Autodesk Fusion 360 part; units mm, degrees
(part 5 of 15)
  spline S28 degree 5 poles (37.7214, 5.5005) (37.7249, 5.5105) (37.7342, 5.5374) (37.7492, 5.5812) (37.7698, 5.6421) (37.7958, 5.72) (37.8238, 5.8051) (37.8515, 5.8904) (37.8788, 5.9759) (37.9057, 6.0616) (37.9322, 6.1474) (37.9584, 6.2335) (37.9843, 6.3197) (38.0098, 6.406) (38.035, 6.4926) (38.0599, 6.5793) (38.0844, 6.6662) (38.1085, 6.7532) (38.1324, 6.8404) (38.1559, 6.9278) (38.1791, 7.0153) (38.202, 7.103) (38.2246, 7.1908) (38.2469, 7.2788) (38.2688, 7.3669) (38.2905, 7.4552) (38.3118, 7.5436) (38.3328, 7.6322) (38.3536, 7.7209) (38.374, 7.8097) (38.3941, 7.8987) (38.414, 7.9878) (38.4335, 8.077) (38.4527, 8.1664) (38.4717, 8.2559) (38.4904, 8.3455) (38.5087, 8.4353) (38.5268, 8.5252) (38.5446, 8.6152) (38.5622, 8.7053) (38.5794, 8.7956) (38.5964, 8.886) (38.613, 8.9764) (38.6262, 9.0489) (38.6359, 9.1034) (38.6423, 9.1397) (38.6455, 9.1578) knots 0.405839 0.405839 0.405839 0.405839 0.405839 0.405839 0.414286 0.428571 0.442857 0.457143 0.471429 0.485714 0.5 0.514286 0.528571 0.542857 0.557143 0.571429 0.585714 0.6 0.614286 0.628571 0.642857 0.657143 0.671429 0.685714 0.7 0.714286 0.728571 0.742857 0.757143 0.771429 0.785714 0.8 0.814286 0.828571 0.842857 0.857143 0.871429 0.885714 0.9 0.914286 0.928571 0.942857 0.957143 0.971429 0.985714 1 1 1 1 1 1
  arc A29 (38.6455, 9.1578) -> (37.5327, 9.873) centre (-2.0032, -52.8695) ccw
  spline S29 degree 5 poles (37.5327, 9.873) (37.5175, 9.8625) (37.4872, 9.8416) (37.4417, 9.8101) (37.3812, 9.7681) (37.3058, 9.7153) (37.2307, 9.6624) (37.1557, 9.6092) (37.081, 9.5558) (37.0065, 9.5022) (36.9323, 9.4484) (36.8583, 9.3944) (36.7845, 9.3402) (36.711, 9.2858) (36.6377, 9.2311) (36.5646, 9.1763) (36.4918, 9.1212) (36.4192, 9.066) (36.3469, 9.0105) (36.2748, 8.9548) (36.203, 8.8989) (36.1314, 8.8427) (36.0601, 8.7864) (35.9891, 8.7298) (35.9183, 8.673) (35.8478, 8.616) (35.7776, 8.5587) (35.7076, 8.5013) (35.6379, 8.4436) (35.5685, 8.3856) (35.4994, 8.3275) (35.4305, 8.2691) (35.3619, 8.2105) (35.2937, 8.1516) (35.2257, 8.0925) (35.158, 8.0332) (35.0907, 7.9736) (35.0236, 7.9138) (34.9569, 7.8537) (34.8904, 7.7934) (34.8243, 7.7328) (34.7586, 7.672) (34.6985, 7.6159) (34.6517, 7.5719) (34.618, 7.54) (34.5974, 7.5204) (34.5898, 7.5131) knots -1 -1 -1 -1 -1 -1 -0.985714 -0.971429 -0.957143 -0.942857 -0.928571 -0.914286 -0.9 -0.885714 -0.871429 -0.857143 -0.842857 -0.828571 -0.814286 -0.8 -0.785714 -0.771429 -0.757143 -0.742857 -0.728571 -0.714286 -0.7 -0.685714 -0.671429 -0.657143 -0.642857 -0.628571 -0.614286 -0.6 -0.585714 -0.571429 -0.557143 -0.542857 -0.528571 -0.514286 -0.5 -0.485714 -0.471429 -0.457143 -0.442857 -0.428571 -0.414286 -0.405839 -0.405839 -0.405839 -0.405839 -0.405839 -0.405839
  arc A30 (34.5898, 7.5131) -> (33.4562, 8.1857) centre (-2.0032, -52.8695) ccw
  spline S30 degree 5 poles (33.4562, 8.1857) (33.4589, 8.1959) (33.4662, 8.2234) (33.4781, 8.2682) (33.4943, 8.3304) (33.5147, 8.41) (33.5366, 8.4969) (33.5581, 8.5839) (33.5792, 8.6711) (33.5999, 8.7585) (33.6203, 8.846) (33.6403, 8.9337) (33.6599, 9.0215) (33.6792, 9.1095) (33.6982, 9.1976) (33.7168, 9.2859) (33.735, 9.3743) (33.7529, 9.4629) (33.7705, 9.5515) (33.7877, 9.6404) (33.8046, 9.7293) (33.8212, 9.8184) (33.8375, 9.9076) (33.8534, 9.997) (33.869, 10.0864) (33.8843, 10.176) (33.8993, 10.2657) (33.9139, 10.3556) (33.9283, 10.4455) (33.9423, 10.5356) (33.956, 10.6257) (33.9695, 10.716) (33.9826, 10.8065) (33.9954, 10.897) (34.0079, 10.9876) (34.0202, 11.0783) (34.0321, 11.1692) (34.0437, 11.2601) (34.0551, 11.3512) (34.0661, 11.4423) (34.0769, 11.5336) (34.0873, 11.6249) (34.0975, 11.7164) (34.1054, 11.7896) (34.1113, 11.8446) (34.1151, 11.8813) (34.117, 11.8996) knots 0.405839 0.405839 0.405839 0.405839 0.405839 0.405839 0.414286 0.428571 0.442857 0.457143 0.471429 0.485714 0.5 0.514286 0.528571 0.542857 0.557143 0.571429 0.585714 0.6 0.614286 0.628571 0.642857 0.657143 0.671429 0.685714 0.7 0.714286 0.728571 0.742857 0.757143 0.771429 0.785714 0.8 0.814286 0.828571 0.842857 0.857143 0.871429 0.885714 0.9 0.914286 0.928571 0.942857 0.957143 0.971429 0.985714 1 1 1 1 1 1
  arc A31 (34.117, 11.8996) -> (32.956, 12.5336) centre (-2.0032, -52.8695) ccw
  spline S31 degree 5 poles (32.956, 12.5336) (32.9416, 12.5221) (32.9128, 12.499) (32.8697, 12.4644) (32.8124, 12.4182) (32.7409, 12.3601) (32.6697, 12.3019) (32.5988, 12.2436) (32.5281, 12.185) (32.4576, 12.1262) (32.3874, 12.0672) (32.3174, 12.0081) (32.2477, 11.9488) (32.1782, 11.8892) (32.109, 11.8295) (32.04, 11.7696) (31.9713, 11.7095) (31.9029, 11.6492) (31.8347, 11.5887) (31.7668, 11.528) (31.6992, 11.4671) (31.6318, 11.406) (31.5647, 11.3447) (31.4979, 11.2832) (31.4313, 11.2215) (31.365, 11.1596) (31.2991, 11.0975) (31.2334, 11.0352) (31.168, 10.9726) (31.1029, 10.9099) (31.0381, 10.847) (30.9736, 10.7838) (30.9093, 10.7204) (30.8455, 10.6569) (30.7819, 10.5931) (30.7186, 10.5291) (30.6557, 10.4648) (30.593, 10.4004) (30.5308, 10.3357) (30.4688, 10.2708) (30.4072, 10.2057) (30.3459, 10.1403) (30.29, 10.0801) (30.2465, 10.0328) (30.2152, 9.9986) (30.196, 9.9776) (30.1889, 9.9698) knots -1 -1 -1 -1 -1 -1 -0.985714 -0.971429 -0.957143 -0.942857 -0.928571 -0.914286 -0.9 -0.885714 -0.871429 -0.857143 -0.842857 -0.828571 -0.814286 -0.8 -0.785714 -0.771429 -0.757143 -0.742857 -0.728571 -0.714286 -0.7 -0.685714 -0.671429 -0.657143 -0.642857 -0.628571 -0.614286 -0.6 -0.585714 -0.571429 -0.557143 -0.542857 -0.528571 -0.514286 -0.5 -0.485714 -0.471429 -0.457143 -0.442857 -0.428571 -0.414286 -0.405839 -0.405839 -0.405839 -0.405839 -0.405839 -0.405839
  arc A32 (30.1889, 9.9698) -> (29.0102, 10.5598) centre (-2.0032, -52.8695) ccw
  spline S32 degree 5 poles (29.0102, 10.5598) (29.0122, 10.5702) (29.0175, 10.5981) (29.0261, 10.6436) (29.0379, 10.7068) (29.0526, 10.7877) (29.0682, 10.8759) (29.0834, 10.9643) (29.0982, 11.0528) (29.1127, 11.1414) (29.1268, 11.2301) (29.1405, 11.319) (29.1538, 11.408) (29.1668, 11.4972) (29.1794, 11.5864) (29.1916, 11.6758) (29.2035, 11.7653) (29.2151, 11.8549) (29.2263, 11.9446) (29.2371, 12.0344) (29.2477, 12.1243) (29.2578, 12.2144) (29.2677, 12.3045) (29.2772, 12.3948) (29.2864, 12.4851) (29.2952, 12.5756) (29.3038, 12.6661) (29.312, 12.7568) (29.3199, 12.8475) (29.3275, 12.9383) (29.3347, 13.0293) (29.3417, 13.1203) (29.3483, 13.2114) (29.3546, 13.3026) (29.3607, 13.3939) (29.3664, 13.4853) (29.3718, 13.5767) (29.3769, 13.6683) (29.3817, 13.7599) (29.3862, 13.8516) (29.3905, 13.9434) (29.3944, 14.0353) (29.398, 14.1272) (29.4007, 14.2009) (29.4026, 14.2561) (29.4038, 14.293) (29.4044, 14.3114) knots 0.405839 0.405839 0.405839 0.405839 0.405839 0.405839 0.414286 0.428571 0.442857 0.457143 0.471429 0.485714 0.5 0.514286 0.528571 0.542857 0.557143 0.571429 0.585714 0.6 0.614286 0.628571 0.642857 0.657143 0.671429 0.685714 0.7 0.714286 0.728571 0.742857 0.757143 0.771429 0.785714 0.8 0.814286 0.828571 0.842857 0.857143 0.871429 0.885714 0.9 0.914286 0.928571 0.942857 0.957143 0.971429 0.985714 1 1 1 1 1 1
  arc A33 (29.4044, 14.3114) -> (28.2011, 14.8609) centre (-2.0032, -52.8695) ccw
  spline S33 degree 5 poles (28.2011, 14.8609) (28.1876, 14.8484) (28.1605, 14.8234) (28.12, 14.7858) (28.0661, 14.7355) (27.999, 14.6726) (27.9321, 14.6094) (27.8655, 14.5461) (27.7992, 14.4827) (27.7331, 14.419) (27.6672, 14.3552) (27.6017, 14.2912) (27.5363, 14.227) (27.4713, 14.1627) (27.4065, 14.0982) (27.342, 14.0335) (27.2778, 13.9687) (27.2138, 13.9036) (27.1501, 13.8384) (27.0867, 13.773) (27.0236, 13.7075) (26.9607, 13.6417) (26.8982, 13.5758) (26.8359, 13.5097) (26.7739, 13.4434) (26.7122, 13.3769) (26.6509, 13.3102) (26.5898, 13.2434) (26.529, 13.1764) (26.4685, 13.1092) (26.4084, 13.0418) (26.3486, 12.9742) (26.289, 12.9064) (26.2298, 12.8384) (26.171, 12.7702) (26.1124, 12.7019) (26.0542, 12.6333) (25.9964, 12.5646) (25.9389, 12.4956) (25.8817, 12.4264) (25.8249, 12.3571) (25.7684, 12.2875) (25.7169, 12.2234) (25.6769, 12.1732) (25.6481, 12.1369) (25.6305, 12.1145) (25.624, 12.1062) knots -1 -1 -1 -1 -1 -1 -0.985714 -0.971429 -0.957143 -0.942857 -0.928571 -0.914286 -0.9 -0.885714 -0.871429 -0.857143 -0.842857 -0.828571 -0.814286 -0.8 -0.785714 -0.771429 -0.757143 -0.742857 -0.728571 -0.714286 -0.7 -0.685714 -0.671429 -0.657143 -0.642857 -0.628571 -0.614286 -0.6 -0.585714 -0.571429 -0.557143 -0.542857 -0.528571 -0.514286 -0.5 -0.485714 -0.471429 -0.457143 -0.442857 -0.428571 -0.414286 -0.405839 -0.405839 -0.405839 -0.405839 -0.405839 -0.405839
  arc A34 (25.624, 12.1062) -> (24.4062, 12.6106) centre (-2.0032, -52.8695) ccw
  spline S34 degree 5 poles (24.4062, 12.6106) (24.4074, 12.6211) (24.4108, 12.6494) (24.4161, 12.6954) (24.4233, 12.7593) (24.4322, 12.841) (24.4415, 12.9301) (24.4504, 13.0193) (24.4588, 13.1086) (24.4669, 13.1981) (24.4746, 13.2876) (24.482, 13.3772) (24.4889, 13.467) (24.4955, 13.5568) (24.5017, 13.6467) (24.5075, 13.7367) (24.513, 13.8268) (24.5182, 13.917) (24.5229, 14.0073) (24.5273, 14.0977) (24.5314, 14.1881) (24.5352, 14.2787) (24.5385, 14.3693) (24.5416, 14.46) (24.5443, 14.5508) (24.5467, 14.6416) (24.5488, 14.7326) (24.5505, 14.8236) (24.5519, 14.9146) (24.553, 15.0058) (24.5537, 15.097) (24.5542, 15.1883) (24.5543, 15.2796) (24.5541, 15.3711) (24.5536, 15.4625) (24.5528, 15.5541) (24.5516, 15.6457) (24.5502, 15.7374) (24.5485, 15.8291) (24.5464, 15.9209) (24.5441, 16.0128) (24.5415, 16.1047) (24.5385, 16.1967) (24.536, 16.2703) (24.5339, 16.3256) (24.5324, 16.3624) (24.5317, 16.3808) knots 0.405839 0.405839 0.405839 0.405839 0.405839 0.405839 0.414286 0.428571 0.442857 0.457143 0.471429 0.485714 0.5 0.514286 0.528571 0.542857 0.557143 0.571429 0.585714 0.6 0.614286 0.628571 0.642857 0.657143 0.671429 0.685714 0.7 0.714286 0.728571 0.742857 0.757143 0.771429 0.785714 0.8 0.814286 0.828571 0.842857 0.857143 0.871429 0.885714 0.9 0.914286 0.928571 0.942857 0.957143 0.971429 0.985714 1 1 1 1 1 1
  arc A35 (24.5317, 16.3808) -> (23.2923, 16.8431) centre (-2.0032, -52.8695) ccw
  spline S35 degree 5 poles (23.2923, 16.8431) (23.2797, 16.8296) (23.2545, 16.8027) (23.2168, 16.7623) (23.1666, 16.7084) (23.1041, 16.6408) (23.042, 16.5731) (22.98, 16.5052) (22.9184, 16.4371) (22.857, 16.3689) (22.7959, 16.3006) (22.735, 16.2321) (22.6745, 16.1634) (22.6142, 16.0946) (22.5542, 16.0256) (22.4944, 15.9565) (22.435, 15.8872) (22.3758, 15.8178) (22.3169, 15.7482) (22.2584, 15.6785) (22.2001, 15.6086) (22.1421, 15.5385) (22.0844, 15.4683) (22.027, 15.3979) (21.9699, 15.3274) (21.9131, 15.2566) (21.8566, 15.1858) (21.8005, 15.1148) (21.7447, 15.0436) (21.6891, 14.9722) (21.634, 14.9007) (21.5791, 14.829) (21.5246, 14.7571) (21.4704, 14.6851) (21.4165, 14.6129) (21.363, 14.5405) (21.3098, 14.468) (21.257, 14.3953) (21.2046, 14.3224) (21.1525, 14.2494) (21.1008, 14.1761) (21.0494, 14.1027) (21.0026, 14.0351) (20.9663, 13.9821) (20.9402, 13.9439) (20.9242, 13.9203) (20.9183, 13.9116) knots -1 -1 -1 -1 -1 -1 -0.985714 -0.971429 -0.957143 -0.942857 -0.928571 -0.914286 -0.9 -0.885714 -0.871429 -0.857143 -0.842857 -0.828571 -0.814286 -0.8 -0.785714 -0.771429 -0.757143 -0.742857 -0.728571 -0.714286 -0.7 -0.685714 -0.671429 -0.657143 -0.642857 -0.628571 -0.614286 -0.6 -0.585714 -0.571429 -0.557143 -0.542857 -0.528571 -0.514286 -0.5 -0.485714 -0.471429 -0.457143 -0.442857 -0.428571 -0.414286 -0.405839 -0.405839 -0.405839 -0.405839 -0.405839 -0.405839
  arc A36 (20.9183, 13.9116) -> (19.6676, 14.3278) centre (-2.0032, -52.8695) ccw
  spline S36 degree 5 poles (19.6676, 14.3278) (19.6681, 14.3384) (19.6694, 14.3668) (19.6715, 14.4131) (19.6741, 14.4773) (19.6771, 14.5594) (19.68, 14.649) (19.6825, 14.7386) (19.6846, 14.8283) (19.6863, 14.9181) (19.6876, 15.0079) (19.6885, 15.0979) (19.689, 15.1879) (19.6892, 15.2779) (19.689, 15.3681) (19.6884, 15.4583) (19.6874, 15.5486) (19.6861, 15.6389) (19.6844, 15.7293) (19.6824, 15.8197) (19.68, 15.9102) (19.6772, 16.0008) (19.6742, 16.0914) (19.6707, 16.1821) (19.667, 16.2729) (19.6629, 16.3637) (19.6584, 16.4545) (19.6537, 16.5454) (19.6486, 16.6363) (19.6431, 16.7273) (19.6374, 16.8184) (19.6313, 16.9095) (19.6249, 17.0006) (19.6182, 17.0918) (19.6112, 17.183) (19.6038, 17.2742) (19.5962, 17.3655) (19.5882, 17.4569) (19.5799, 17.5483) (19.5713, 17.6397) (19.5625, 17.7312) (19.5533, 17.8226) (19.5438, 17.9142) (19.536, 17.9874) (19.53, 18.0424) (19.5259, 18.079) (19.5238, 18.0974) knots 0.405839 0.405839 0.405839 0.405839 0.405839 0.405839 0.414286 0.428571 0.442857 0.457143 0.471429 0.485714 0.5 0.514286 0.528571 0.542857 0.557143 0.571429 0.585714 0.6 0.614286 0.628571 0.642857 0.657143 0.671429 0.685714 0.7 0.714286 0.728571 0.742857 0.757143 0.771429 0.785714 0.8 0.814286 0.828571 0.842857 0.857143 0.871429 0.885714 0.9 0.914286 0.928571 0.942857 0.957143 0.971429 0.985714 1 1 1 1 1 1
  arc A37 (19.5238, 18.0974) -> (18.2546, 18.47) centre (-2.0032, -52.8695) ccw
  spline S37 degree 5 poles (18.2546, 18.47) (18.243, 18.4557) (18.2198, 18.4271) (18.185, 18.3841) (18.1388, 18.3267) (18.0814, 18.2548) (18.0242, 18.1828) (17.9672, 18.1107) (17.9106, 18.0384) (17.8542, 17.966) (17.7982, 17.8935) (17.7424, 17.8208) (17.6868, 17.748) (17.6316, 17.6751) (17.5767, 17.602) (17.522, 17.5288) (17.4677, 17.4555) (17.4136, 17.382) (17.3598, 17.3084) (17.3064, 17.2346) (17.2532, 17.1607) (17.2004, 17.0867) (17.1478, 17.0126) (17.0956, 16.9383) (17.0437, 16.8638) (16.9921, 16.7892) (16.9409, 16.7145) (16.8899, 16.6397) (16.8393, 16.5647) (16.789, 16.4895) (16.7391, 16.4143) (16.6895, 16.3388) (16.6402, 16.2633) (16.5913, 16.1876) (16.5427, 16.1117) (16.4945, 16.0357) (16.4466, 15.9596) (16.3991, 15.8833) (16.352, 15.8068) (16.3053, 15.7303) (16.2589, 15.6535) (16.213, 15.5766) (16.1711, 15.5059) (16.1386, 15.4504) (16.1153, 15.4104) (16.101, 15.3858) (16.0958, 15.3766) knots -1 -1 -1 -1 -1 -1 -0.985714 -0.971429 -0.957143 -0.942857 -0.928571 -0.914286 -0.9 -0.885714 -0.871429 -0.857143 -0.842857 -0.828571 -0.814286 -0.8 -0.785714 -0.771429 -0.757143 -0.742857 -0.728571 -0.714286 -0.7 -0.685714 -0.671429 -0.657143 -0.642857 -0.628571 -0.614286 -0.6 -0.585714 -0.571429 -0.557143 -0.542857 -0.528571 -0.514286 -0.5 -0.485714 -0.471429 -0.457143 -0.442857 -0.428571 -0.414286 -0.405839 -0.405839 -0.405839 -0.405839 -0.405839 -0.405839
  arc A38 (16.0958, 15.3766) -> (14.8186, 15.7026) centre (-2.0032, -52.8695) ccw
  spline S38 degree 5 poles (14.8186, 15.7026) (14.8183, 15.7132) (14.8176, 15.7416) (14.8163, 15.7879) (14.8144, 15.8522) (14.8116, 15.9343) (14.8081, 16.0238) (14.8041, 16.1134) (14.7998, 16.203) (14.7951, 16.2927) (14.79, 16.3824) (14.7845, 16.4722) (14.7786, 16.562) (14.7723, 16.6518) (14.7657, 16.7417) (14.7586, 16.8317) (14.7513, 16.9216) (14.7435, 17.0116) (14.7354, 17.1017) (14.7269, 17.1918) (14.718, 17.2819) (14.7089, 17.372) (14.6993, 17.4622) (14.6894, 17.5524) (14.6792, 17.6426) (14.6686, 17.7329) (14.6577, 17.8232) (14.6465, 17.9135) (14.6349, 18.0039) (14.623, 18.0942) (14.6108, 18.1846) (14.5982, 18.2751) (14.5853, 18.3655) (14.5721, 18.456) (14.5586, 18.5465) (14.5448, 18.637) (14.5306, 18.7275) (14.5162, 18.818) (14.5014, 18.9086) (14.4863, 18.9992) (14.4709, 19.0897) (14.4552, 19.1804) (14.4392, 19.271) (14.4262, 19.3435) (14.4163, 19.3979) (14.4096, 19.4341) (14.4063, 19.4523) knots 0.405839 0.405839 0.405839 0.405839 0.405839 0.405839 0.414286 0.428571 0.442857 0.457143 0.471429 0.485714 0.5 0.514286 0.528571 0.542857 0.557143 0.571429 0.585714 0.6 0.614286 0.628571 0.642857 0.657143 0.671429 0.685714 0.7 0.714286 0.728571 0.742857 0.757143 0.771429 0.785714 0.8 0.814286 0.828571 0.842857 0.857143 0.871429 0.885714 0.9 0.914286 0.928571 0.942857 0.957143 0.971429 0.985714 1 1 1 1 1 1
  arc A39 (14.4063, 19.4523) -> (13.1137, 19.7334) centre (-2.0032, -52.8695) ccw
  spline S39 degree 5 poles (13.1137, 19.7334) (13.1031, 19.7183) (13.082, 19.6881) (13.0504, 19.6428) (13.0084, 19.5822) (12.9562, 19.5064) (12.9043, 19.4305) (12.8527, 19.3545) (12.8014, 19.2784) (12.7503, 19.2022) (12.6995, 19.1258) (12.6491, 19.0493) (12.5989, 18.9728) (12.549, 18.8961) (12.4994, 18.8193) (12.4501, 18.7423) (12.4011, 18.6653) (12.3524, 18.5882) (12.3041, 18.5109) (12.256, 18.4335) (12.2083, 18.356) (12.1608, 18.2784) (12.1137, 18.2007) (12.0669, 18.1229) (12.0205, 18.0449) (11.9743, 17.9669) (11.9285, 17.8887) (11.883, 17.8104) (11.8379, 17.732) (11.7931, 17.6534) (11.7487, 17.5748) (11.7046, 17.496) (11.6608, 17.4171) (11.6174, 17.3381) (11.5744, 17.259) (11.5317, 17.1798) (11.4894, 17.1004) (11.4475, 17.0209) (11.406, 16.9413) (11.3648, 16.8616) (11.324, 16.7817) (11.2837, 16.7018) (11.2469, 16.6282) (11.2185, 16.5706) (11.1981, 16.529) (11.1856, 16.5034) (11.181, 16.4939) knots -1 -1 -1 -1 -1 -1 -0.985714 -0.971429 -0.957143 -0.942857 -0.928571 -0.914286 -0.9 -0.885714 -0.871429 -0.857143 -0.842857 -0.828571 -0.814286 -0.8 -0.785714 -0.771429 -0.757143 -0.742857 -0.728571 -0.714286 -0.7 -0.685714 -0.671429 -0.657143 -0.642857 -0.628571 -0.614286 -0.6 -0.585714 -0.571429 -0.557143 -0.542857 -0.528571 -0.514286 -0.5 -0.485714 -0.471429 -0.457143 -0.442857 -0.428571 -0.414286 -0.405839 -0.405839 -0.405839 -0.405839 -0.405839 -0.405839
  arc A40 (11.181, 16.4939) -> (9.8838, 16.7279) centre (-2.0032, -52.8695) ccw
  spline S40 degree 5 poles (9.8838, 16.7279) (9.8828, 16.7385) (9.8801, 16.7668) (9.8755, 16.8129) (9.869, 16.8768) (9.8603, 16.9586) (9.8504, 17.0476) (9.8401, 17.1367) (9.8294, 17.2257) (9.8183, 17.3149) (9.8068, 17.404) (9.7949, 17.4931) (9.7827, 17.5823) (9.77, 17.6714) (9.7569, 17.7606) (9.7435, 17.8498) (9.7297, 17.9391) (9.7156, 18.0283) (9.701, 18.1175) (9.6861, 18.2068) (9.6709, 18.296) (9.6553, 18.3853) (9.6394, 18.4745) (9.6231, 18.5638) (9.6064, 18.6531) (9.5894, 18.7424) (9.5721, 18.8317) (9.5545, 18.921) (9.5365, 19.0102) (9.5181, 19.0995) (9.4995, 19.1888) (9.4805, 19.2781) (9.4612, 19.3674) (9.4416, 19.4567) (9.4217, 19.546) (9.4014, 19.6353) (9.3808, 19.7246) (9.3599, 19.8138) (9.3387, 19.9031) (9.3172, 19.9924) (9.2954, 20.0817) (9.2733, 20.1709) (9.2509, 20.2602) (9.2327, 20.3316) (9.219, 20.3851) (9.2097, 20.4208) (9.2051, 20.4386) knots 0.405839 0.405839 0.405839 0.405839 0.405839 0.405839 0.414286 0.428571 0.442857 0.457143 0.471429 0.485714 0.5 0.514286 0.528571 0.542857 0.557143 0.571429 0.585714 0.6 0.614286 0.628571 0.642857 0.657143 0.671429 0.685714 0.7 0.714286 0.728571 0.742857 0.757143 0.771429 0.785714 0.8 0.814286 0.828571 0.842857 0.857143 0.871429 0.885714 0.9 0.914286 0.928571 0.942857 0.957143 0.971429 0.985714 1 1 1 1 1 1
  arc A41 (9.2051, 20.4386) -> (7.8958, 20.6269) centre (-2.0032, -52.8695) ccw
  spline S41 degree 5 poles (7.8958, 20.6269) (7.8863, 20.6111) (7.8674, 20.5794) (7.8391, 20.5319) (7.8015, 20.4685) (7.7549, 20.3892) (7.7085, 20.3098) (7.6624, 20.2303) (7.6167, 20.1507) (7.5712, 20.071) (7.526, 19.9913) (7.4811, 19.9114) (7.4365, 19.8314) (7.3922, 19.7514) (7.3482, 19.6712) (7.3046, 19.591) (7.2612, 19.5106) (7.2181, 19.4302) (7.1754, 19.3497) (7.133, 19.2691) (7.0909, 19.1884) (7.0491, 19.1076) (7.0077, 19.0267) (6.9665, 18.9458) (6.9258, 18.8647) (6.8853, 18.7835) (6.8452, 18.7023) (6.8054, 18.6209) (6.766, 18.5395) (6.7269, 18.458) (6.6882, 18.3764) (6.6498, 18.2946) (6.6118, 18.2128) (6.5742, 18.1309) (6.5369, 18.0489) (6.5, 17.9669) (6.4634, 17.8847) (6.4273, 17.8024) (6.3915, 17.72) (6.3562, 17.6376) (6.3212, 17.555) (6.2866, 17.4724) (6.2553, 17.3964) (6.231, 17.3369) (6.2136, 17.2939) (6.203, 17.2675) (6.1991, 17.2577) knots -1 -1 -1 -1 -1 -1 -0.985714 -0.971429 -0.957143 -0.942857 -0.928571 -0.914286 -0.9 -0.885714 -0.871429 -0.857143 -0.842857 -0.828571 -0.814286 -0.8 -0.785714 -0.771429 -0.757143 -0.742857 -0.728571 -0.714286 -0.7 -0.685714 -0.671429 -0.657143 -0.642857 -0.628571 -0.614286 -0.6 -0.585714 -0.571429 -0.557143 -0.542857 -0.528571 -0.514286 -0.5 -0.485714 -0.471429 -0.457143 -0.442857 -0.428571 -0.414286 -0.405839 -0.405839 -0.405839 -0.405839 -0.405839 -0.405839
  arc A42 (6.1991, 17.2577) -> (4.8885, 17.3986) centre (-2.0032, -52.8695) ccw
  spline S42 degree 5 poles (4.8885, 17.3986) (4.8868, 17.409) (4.882, 17.4371) (4.8742, 17.4828) (4.8631, 17.5461) (4.8486, 17.627) (4.8324, 17.7151) (4.8158, 17.8032) (4.7988, 17.8913) (4.7813, 17.9794) (4.7635, 18.0674) (4.7453, 18.1555) (4.7267, 18.2436) (4.7077, 18.3316) (4.6883, 18.4196) (4.6685, 18.5077) (4.6484, 18.5957) (4.6279, 18.6836) (4.6071, 18.7716) (4.5858, 18.8596) (4.5643, 18.9475) (4.5423, 19.0354) (4.5201, 19.1233) (4.4974, 19.2112) (4.4745, 19.2991) (4.4512, 19.3869) (4.4275, 19.4747) (4.4035, 19.5626) (4.3792, 19.6503) (4.3546, 19.7381) (4.3296, 19.8258) (4.3043, 19.9135) (4.2787, 20.0012) (4.2527, 20.0889) (4.2265, 20.1765) (4.1999, 20.2641) (4.173, 20.3517) (4.1458, 20.4393) (4.1183, 20.5268) (4.0905, 20.6143) (4.0624, 20.7018) (4.034, 20.7893) (4.0052, 20.8767) (3.982, 20.9466) (3.9645, 20.999) (3.9527, 21.034) (3.9468, 21.0514) knots 0.405839 0.405839 0.405839 0.405839 0.405839 0.405839 0.414286 0.428571 0.442857 0.457143 0.471429 0.485714 0.5 0.514286 0.528571 0.542857 0.557143 0.571429 0.585714 0.6 0.614286 0.628571 0.642857 0.657143 0.671429 0.685714 0.7 0.714286 0.728571 0.742857 0.757143 0.771429 0.785714 0.8 0.814286 0.828571 0.842857 0.857143 0.871429 0.885714 0.9 0.914286 0.928571 0.942857 0.957143 0.971429 0.985714 1 1 1 1 1 1
  arc A43 (3.9468, 21.0514) -> (2.6274, 21.1458) centre (-2.0032, -52.8695) ccw
  spline S43 degree 5 poles (2.6274, 21.1458) (2.6191, 21.1294) (2.6024, 21.0964) (2.5776, 21.0471) (2.5447, 20.9812) (2.5038, 20.8987) (2.4632, 20.8162) (2.4229, 20.7336) (2.383, 20.6509) (2.3433, 20.5682) (2.3039, 20.4854) (2.2648, 20.4025) (2.226, 20.3196) (2.1876, 20.2366) (2.1494, 20.1535) (2.1116, 20.0704) (2.074, 19.9871) (2.0368, 19.9039) (2, 19.8205) (1.9634, 19.7371) (1.9272, 19.6536) (1.8913, 19.57) (1.8557, 19.4864) (1.8205, 19.4027) (1.7855, 19.3189) (1.751, 19.2351) (1.7168, 19.1512) (1.6829, 19.0672) (1.6494, 18.9832) (1.6162, 18.899) (1.5834, 18.8149) (1.551, 18.7306) (1.5189, 18.6463) (1.4872, 18.5619) (1.4559, 18.4775) (1.4249, 18.393) (1.3943, 18.3084) (1.3641, 18.2238) (1.3344, 18.1391) (1.305, 18.0543) (1.276, 17.9694) (1.2474, 17.8845) (1.2215, 17.8065) (1.2016, 17.7454) (1.1873, 17.7013) (1.1786, 17.6743) (1.1754, 17.6642) knots -1 -1 -1 -1 -1 -1 -0.985714 -0.971429 -0.957143 -0.942857 -0.928571 -0.914286 -0.9 -0.885714 -0.871429 -0.857143 -0.842857 -0.828571 -0.814286 -0.8 -0.785714 -0.771429 -0.757143 -0.742857 -0.728571 -0.714286 -0.7 -0.685714 -0.671429 -0.657143 -0.642857 -0.628571 -0.614286 -0.6 -0.585714 -0.571429 -0.557143 -0.542857 -0.528571 -0.514286 -0.5 -0.485714 -0.471429 -0.457143 -0.442857 -0.428571 -0.414286 -0.405839 -0.405839 -0.405839 -0.405839 -0.405839 -0.405839
  arc A44 (1.1754, 17.6642) -> (-0.1419, 17.7112) centre (-2.0032, -52.8695) ccw
  spline S44 degree 5 poles (-0.1419, 17.7112) (-0.1444, 17.7215) (-0.1511, 17.7491) (-0.1622, 17.7941) (-0.1778, 17.8565) (-0.198, 17.9362) (-0.2205, 18.0229) (-0.2433, 18.1096) (-0.2666, 18.1962) (-0.2903, 18.2829) (-0.3143, 18.3694) (-0.3388, 18.456) (-0.3636, 18.5425) (-0.3889, 18.6289) (-0.4145, 18.7154) (-0.4405, 18.8018) (-0.4668, 18.8881) (-0.4935, 18.9744) (-0.5206, 19.0607) (-0.548, 19.1469) (-0.5758, 19.233) (-0.604, 19.3192) (-0.6325, 19.4053) (-0.6613, 19.4913) (-0.6905, 19.5773) (-0.72, 19.6633) (-0.7498, 19.7492) (-0.78, 19.8351) (-0.8105, 19.9209) (-0.8414, 20.0067) (-0.8726, 20.0924) (-0.904, 20.1781) (-0.9359, 20.2637) (-0.968, 20.3493) (-1.0004, 20.4348) (-1.0332, 20.5203) (-1.0663, 20.6058) (-1.0996, 20.6912) (-1.1333, 20.7765) (-1.1673, 20.8618) (-1.2016, 20.9471) (-1.2362, 21.0323) (-1.2711, 21.1174) (-1.2992, 21.1855) (-1.3205, 21.2366) (-1.3347, 21.2706) (-1.3418, 21.2876) knots 0.405839 0.405839 0.405839 0.405839 0.405839 0.405839 0.414286 0.428571 0.442857 0.457143 0.471429 0.485714 0.5 0.514286 0.528571 0.542857 0.557143 0.571429 0.585714 0.6 0.614286 0.628571 0.642857 0.657143 0.671429 0.685714 0.7 0.714286 0.728571 0.742857 0.757143 0.771429 0.785714 0.8 0.814286 0.828571 0.842857 0.857143 0.871429 0.885714 0.9 0.914286 0.928571 0.942857 0.957143 0.971429 0.985714 1 1 1 1 1 1
  arc A45 (-1.3418, 21.2876) -> (-2.6646, 21.2876) centre (-2.0032, -52.8695) ccw
  spline S45 degree 5 poles (-2.6646, 21.2876) (-2.6717, 21.2706) (-2.686, 21.2366) (-2.7072, 21.1855) (-2.7354, 21.1174) (-2.7702, 21.0323) (-2.8048, 20.9471) (-2.8391, 20.8618) (-2.8731, 20.7765) (-2.9068, 20.6912) (-2.9402, 20.6058) (-2.9732, 20.5203) (-3.006, 20.4348) (-3.0384, 20.3493) (-3.0706, 20.2637) (-3.1024, 20.1781) (-3.1339, 20.0924) (-3.165, 20.0067) (-3.1959, 19.9209) (-3.2264, 19.8351) (-3.2566, 19.7492) (-3.2864, 19.6633) (-3.316, 19.5773) (-3.3451, 19.4913) (-3.374, 19.4053) (-3.4025, 19.3192) (-3.4306, 19.233) (-3.4584, 19.1469) (-3.4858, 19.0607) (-3.5129, 18.9744) (-3.5396, 18.8881) (-3.566, 18.8018) (-3.592, 18.7154) (-3.6176, 18.6289) (-3.6428, 18.5425) (-3.6676, 18.456) (-3.6921, 18.3694) (-3.7162, 18.2829) (-3.7398, 18.1962) (-3.7631, 18.1096) (-3.786, 18.0229) (-3.8084, 17.9362) (-3.8287, 17.8565) (-3.8442, 17.7941) (-3.8553, 17.7491) (-3.862, 17.7215) (-3.8645, 17.7112) knots -1 -1 -1 -1 -1 -1 -0.985714 -0.971429 -0.957143 -0.942857 -0.928571 -0.914286 -0.9 -0.885714 -0.871429 -0.857143 -0.842857 -0.828571 -0.814286 -0.8 -0.785714 -0.771429 -0.757143 -0.742857 -0.728571 -0.714286 -0.7 -0.685714 -0.671429 -0.657143 -0.642857 -0.628571 -0.614286 -0.6 -0.585714 -0.571429 -0.557143 -0.542857 -0.528571 -0.514286 -0.5 -0.485714 -0.471429 -0.457143 -0.442857 -0.428571 -0.414286 -0.405839 -0.405839 -0.405839 -0.405839 -0.405839 -0.405839
  arc A46 (-3.8645, 17.7112) -> (-5.1818, 17.6642) centre (-2.0032, -52.8695) ccw
  spline S46 degree 5 poles (-5.1818, 17.6642) (-5.185, 17.6743) (-5.1937, 17.7013) (-5.208, 17.7454) (-5.228, 17.8065) (-5.2538, 17.8845) (-5.2824, 17.9694) (-5.3114, 18.0543) (-5.3408, 18.1391) (-5.3706, 18.2238) (-5.4008, 18.3084) (-5.4313, 18.393) (-5.4623, 18.4775) (-5.4936, 18.5619) (-5.5253, 18.6463) (-5.5574, 18.7306) (-5.5898, 18.8149) (-5.6227, 18.899) (-5.6558, 18.9832) (-5.6893, 19.0672) (-5.7232, 19.1512) (-5.7574, 19.2351) (-5.792, 19.3189) (-5.8269, 19.4027) (-5.8621, 19.4864) (-5.8977, 19.57) (-5.9336, 19.6536) (-5.9698, 19.7371) (-6.0064, 19.8205) (-6.0433, 19.9039) (-6.0805, 19.9871) (-6.118, 20.0704) (-6.1558, 20.1535) (-6.194, 20.2366) (-6.2325, 20.3196) (-6.2712, 20.4025) (-6.3103, 20.4854) (-6.3497, 20.5682) (-6.3894, 20.6509) (-6.4294, 20.7336) (-6.4697, 20.8162) (-6.5102, 20.8987) (-6.5511, 20.9812) (-6.584, 21.0471) (-6.6089, 21.0964) (-6.6255, 21.1294) (-6.6338, 21.1458) knots 0.405839 0.405839 0.405839 0.405839 0.405839 0.405839 0.414286 0.428571 0.442857 0.457143 0.471429 0.485714 0.5 0.514286 0.528571 0.542857 0.557143 0.571429 0.585714 0.6 0.614286 0.628571 0.642857 0.657143 0.671429 0.685714 0.7 0.714286 0.728571 0.742857 0.757143 0.771429 0.785714 0.8 0.814286 0.828571 0.842857 0.857143 0.871429 0.885714 0.9 0.914286 0.928571 0.942857 0.957143 0.971429 0.985714 1 1 1 1 1 1
  arc A47 (-6.6338, 21.1458) -> (-7.9532, 21.0514) centre (-2.0032, -52.8695) ccw
  spline S47 degree 5 poles (-7.9532, 21.0514) (-7.9591, 21.034) (-7.9709, 20.999) (-7.9884, 20.9466) (-8.0117, 20.8767) (-8.0404, 20.7893) (-8.0688, 20.7018) (-8.0969, 20.6143) (-8.1247, 20.5268) (-8.1522, 20.4393) (-8.1794, 20.3517) (-8.2063, 20.2641) (-8.2329, 20.1765) (-8.2592, 20.0889) (-8.2851, 20.0012) (-8.3107, 19.9135) (-8.336, 19.8258) (-8.361, 19.7381) (-8.3856, 19.6503) (-8.41, 19.5626) (-8.4339, 19.4747) (-8.4576, 19.3869) (-8.4809, 19.2991) (-8.5039, 19.2112) (-8.5265, 19.1233) (-8.5488, 19.0354) (-8.5707, 18.9475) (-8.5923, 18.8596) (-8.6135, 18.7716) (-8.6343, 18.6836) (-8.6548, 18.5957) (-8.675, 18.5077) (-8.6947, 18.4196) (-8.7141, 18.3316) (-8.7331, 18.2436) (-8.7517, 18.1555) (-8.7699, 18.0674) (-8.7878, 17.9794) (-8.8052, 17.8913) (-8.8222, 17.8032) (-8.8388, 17.7151) (-8.855, 17.627) (-8.8695, 17.5461) (-8.8806, 17.4828) (-8.8884, 17.4371) (-8.8932, 17.409) (-8.895, 17.3986) knots -1 -1 -1 -1 -1 -1 -0.985714 -0.971429 -0.957143 -0.942857 -0.928571 -0.914286 -0.9 -0.885714 -0.871429 -0.857143 -0.842857 -0.828571 -0.814286 -0.8 -0.785714 -0.771429 -0.757143 -0.742857 -0.728571 -0.714286 -0.7 -0.685714 -0.671429 -0.657143 -0.642857 -0.628571 -0.614286 -0.6 -0.585714 -0.571429 -0.557143 -0.542857 -0.528571 -0.514286 -0.5 -0.485714 -0.471429 -0.457143 -0.442857 -0.428571 -0.414286 -0.405839 -0.405839 -0.405839 -0.405839 -0.405839 -0.405839
  arc A48 (-8.895, 17.3986) -> (-10.2055, 17.2577) centre (-2.0032, -52.8695) ccw
  spline S48 degree 5 poles (-10.2055, 17.2577) (-10.2095, 17.2675) (-10.2201, 17.2939) (-10.2374, 17.3369) (-10.2617, 17.3964) (-10.2931, 17.4724) (-10.3276, 17.555) (-10.3626, 17.6376) (-10.398, 17.72) (-10.4337, 17.8024) (-10.4699, 17.8847) (-10.5064, 17.9669) (-10.5433, 18.0489) (-10.5806, 18.1309) (-10.6182, 18.2128) (-10.6562, 18.2946) (-10.6946, 18.3764) (-10.7333, 18.458) (-10.7724, 18.5395) (-10.8118, 18.6209) (-10.8516, 18.7023) (-10.8917, 18.7835) (-10.9322, 18.8647) (-10.973, 18.9458) (-11.0141, 19.0267) (-11.0555, 19.1076) (-11.0973, 19.1884) (-11.1394, 19.2691) (-11.1818, 19.3497) (-11.2246, 19.4302) (-11.2676, 19.5106) (-11.311, 19.591) (-11.3547, 19.6712) (-11.3986, 19.7514) (-11.4429, 19.8314) (-11.4875, 19.9114) (-11.5324, 19.9913) (-11.5776, 20.071) (-11.6231, 20.1507) (-11.6689, 20.2303) (-11.7149, 20.3098) (-11.7613, 20.3892) (-11.808, 20.4685) (-11.8455, 20.5319) (-11.8738, 20.5794) (-11.8927, 20.6111) (-11.9022, 20.6269) knots 0.405839 0.405839 0.405839 0.405839 0.405839 0.405839 0.414286 0.428571 0.442857 0.457143 0.471429 0.485714 0.5 0.514286 0.528571 0.542857 0.557143 0.571429 0.585714 0.6 0.614286 0.628571 0.642857 0.657143 0.671429 0.685714 0.7 0.714286 0.728571 0.742857 0.757143 0.771429 0.785714 0.8 0.814286 0.828571 0.842857 0.857143 0.871429 0.885714 0.9 0.914286 0.928571 0.942857 0.957143 0.971429 0.985714 1 1 1 1 1 1
  arc A49 (-11.9022, 20.6269) -> (-13.2115, 20.4386) centre (-2.0032, -52.8695) ccw
  spline S49 degree 5 poles (-13.2115, 20.4386) (-13.2162, 20.4208) (-13.2254, 20.3851) (-13.2392, 20.3316) (-13.2573, 20.2602) (-13.2798, 20.1709) (-13.3019, 20.0817) (-13.3237, 19.9924) (-13.3452, 19.9031) (-13.3664, 19.8138) (-13.3873, 19.7246) (-13.4078, 19.6353) (-13.4281, 19.546) (-13.448, 19.4567) (-13.4676, 19.3674) (-13.4869, 19.2781) (-13.5059, 19.1888) (-13.5246, 19.0995) (-13.5429, 19.0102) (-13.5609, 18.921) (-13.5785, 18.8317) (-13.5959, 18.7424) (-13.6128, 18.6531) (-13.6295, 18.5638) (-13.6458, 18.4745) (-13.6617, 18.3853) (-13.6773, 18.296) (-13.6926, 18.2068) (-13.7075, 18.1175) (-13.722, 18.0283) (-13.7362, 17.9391) (-13.7499, 17.8498) (-13.7634, 17.7606) (-13.7764, 17.6714) (-13.7891, 17.5823) (-13.8014, 17.4931) (-13.8133, 17.404) (-13.8248, 17.3149) (-13.8359, 17.2257) (-13.8466, 17.1367) (-13.8569, 17.0476) (-13.8667, 16.9586) (-13.8754, 16.8768) (-13.882, 16.8129) (-13.8865, 16.7668) (-13.8893, 16.7385) (-13.8903, 16.7279) knots -1 -1 -1 -1 -1 -1 -0.985714 -0.971429 -0.957143 -0.942857 -0.928571 -0.914286 -0.9 -0.885714 -0.871429 -0.857143 -0.842857 -0.828571 -0.814286 -0.8 -0.785714 -0.771429 -0.757143 -0.742857 -0.728571 -0.714286 -0.7 -0.685714 -0.671429 -0.657143 -0.642857 -0.628571 -0.614286 -0.6 -0.585714 -0.571429 -0.557143 -0.542857 -0.528571 -0.514286 -0.5 -0.485714 -0.471429 -0.457143 -0.442857 -0.428571 -0.414286 -0.405839 -0.405839 -0.405839 -0.405839 -0.405839 -0.405839
  arc A50 (-13.8903, 16.7279) -> (-15.1874, 16.4939) centre (-2.0032, -52.8695) ccw
  spline S50 degree 5 poles (-15.1874, 16.4939) (-15.1921, 16.5034) (-15.2045, 16.529) (-15.2249, 16.5706) (-15.2534, 16.6282) (-15.2901, 16.7018) (-15.3305, 16.7817) (-15.3712, 16.8616) (-15.4124, 16.9413) (-15.4539, 17.0209) (-15.4958, 17.1004) (-15.5381, 17.1798) (-15.5808, 17.259) (-15.6238, 17.3381) (-15.6672, 17.4171) (-15.711, 17.496) (-15.7551, 17.5748) (-15.7995, 17.6534) (-15.8443, 17.732) (-15.8895, 17.8104) (-15.9349, 17.8887) (-15.9808, 17.9669) (-16.0269, 18.0449) (-16.0734, 18.1229) (-16.1202, 18.2007) (-16.1673, 18.2784) (-16.2147, 18.356) (-16.2624, 18.4335) (-16.3105, 18.5109) (-16.3589, 18.5882) (-16.4076, 18.6653) (-16.4565, 18.7423) (-16.5058, 18.8193) (-16.5554, 18.8961) (-16.6053, 18.9728) (-16.6555, 19.0493) (-16.706, 19.1258) (-16.7567, 19.2022) (-16.8078, 19.2784) (-16.8591, 19.3545) (-16.9108, 19.4305) (-16.9627, 19.5064) (-17.0149, 19.5822) (-17.0568, 19.6428) (-17.0884, 19.6881) (-17.1096, 19.7183) (-17.1202, 19.7334) knots 0.405839 0.405839 0.405839 0.405839 0.405839 0.405839 0.414286 0.428571 0.442857 0.457143 0.471429 0.485714 0.5 0.514286 0.528571 0.542857 0.557143 0.571429 0.585714 0.6 0.614286 0.628571 0.642857 0.657143 0.671429 0.685714 0.7 0.714286 0.728571 0.742857 0.757143 0.771429 0.785714 0.8 0.814286 0.828571 0.842857 0.857143 0.871429 0.885714 0.9 0.914286 0.928571 0.942857 0.957143 0.971429 0.985714 1 1 1 1 1 1
  arc A51 (-17.1202, 19.7334) -> (-18.4127, 19.4523) centre (-2.0032, -52.8695) ccw
  spline S51 degree 5 poles (-18.4127, 19.4523) (-18.4161, 19.4341) (-18.4227, 19.3979) (-18.4326, 19.3435) (-18.4457, 19.271) (-18.4617, 19.1804) (-18.4774, 19.0897) (-18.4927, 18.9992) (-18.5078, 18.9086) (-18.5226, 18.818) (-18.537, 18.7275) (-18.5512, 18.637) (-18.565, 18.5465) (-18.5786, 18.456) (-18.5918, 18.3655) (-18.6046, 18.2751) (-18.6172, 18.1846) (-18.6294, 18.0942) (-18.6413, 18.0039) (-18.6529, 17.9135) (-18.6641, 17.8232) (-18.6751, 17.7329) (-18.6856, 17.6426) (-18.6959, 17.5524) (-18.7057, 17.4622) (-18.7153, 17.372) (-18.7245, 17.2819) (-18.7333, 17.1918) (-18.7418, 17.1017) (-18.7499, 17.0116) (-18.7577, 16.9216) (-18.7651, 16.8317) (-18.7721, 16.7417) (-18.7788, 16.6518) (-18.785, 16.562) (-18.7909, 16.4722) (-18.7964, 16.3824) (-18.8015, 16.2927) (-18.8063, 16.203) (-18.8106, 16.1134) (-18.8145, 16.0238) (-18.818, 15.9343) (-18.8208, 15.8522) (-18.8228, 15.7879) (-18.824, 15.7416) (-18.8248, 15.7132) (-18.825, 15.7026) knots -1 -1 -1 -1 -1 -1 -0.985714 -0.971429 -0.957143 -0.942857 -0.928571 -0.914286 -0.9 -0.885714 -0.871429 -0.857143 -0.842857 -0.828571 -0.814286 -0.8 -0.785714 -0.771429 -0.757143 -0.742857 -0.728571 -0.714286 -0.7 -0.685714 -0.671429 -0.657143 -0.642857 -0.628571 -0.614286 -0.6 -0.585714 -0.571429 -0.557143 -0.542857 -0.528571 -0.514286 -0.5 -0.485714 -0.471429 -0.457143 -0.442857 -0.428571 -0.414286 -0.405839 -0.405839 -0.405839 -0.405839 -0.405839 -0.405839
  arc A52 (-18.825, 15.7026) -> (-20.1022, 15.3766) centre (-2.0032, -52.8695) ccw
  spline S52 degree 5 poles (-20.1022, 15.3766) (-20.1075, 15.3858) (-20.1217, 15.4104) (-20.145, 15.4504) (-20.1775, 15.5059) (-20.2194, 15.5766) (-20.2654, 15.6535) (-20.3117, 15.7303) (-20.3585, 15.8068) (-20.4056, 15.8833) (-20.4531, 15.9596) (-20.5009, 16.0357) (-20.5491, 16.1117) (-20.5977, 16.1876) (-20.6466, 16.2633) (-20.6959, 16.3388) (-20.7455, 16.4143) (-20.7954, 16.4895) (-20.8457, 16.5647) (-20.8963, 16.6397) (-20.9473, 16.7145) (-20.9985, 16.7892) (-21.0501, 16.8638) (-21.102, 16.9383) (-21.1543, 17.0126) (-21.2068, 17.0867) (-21.2597, 17.1607) (-21.3128, 17.2346) (-21.3663, 17.3084) (-21.42, 17.382) (-21.4741, 17.4555) (-21.5284, 17.5288) (-21.5831, 17.602) (-21.638, 17.6751) (-21.6933, 17.748) (-21.7488, 17.8208) (-21.8046, 17.8935) (-21.8607, 17.966) (-21.917, 18.0384) (-21.9737, 18.1107) (-22.0306, 18.1828) (-22.0878, 18.2548) (-22.1453, 18.3267) (-22.1914, 18.3841) (-22.2262, 18.4271) (-22.2494, 18.4557) (-22.2611, 18.47) knots 0.405839 0.405839 0.405839 0.405839 0.405839 0.405839 0.414286 0.428571 0.442857 0.457143 0.471429 0.485714 0.5 0.514286 0.528571 0.542857 0.557143 0.571429 0.585714 0.6 0.614286 0.628571 0.642857 0.657143 0.671429 0.685714 0.7 0.714286 0.728571 0.742857 0.757143 0.771429 0.785714 0.8 0.814286 0.828571 0.842857 0.857143 0.871429 0.885714 0.9 0.914286 0.928571 0.942857 0.957143 0.971429 0.985714 1 1 1 1 1 1
  arc A53 (-22.2611, 18.47) -> (-23.5303, 18.0974) centre (-2.0032, -52.8695) ccw
  spline S53 degree 5 poles (-23.5303, 18.0974) (-23.5323, 18.079) (-23.5364, 18.0424) (-23.5424, 17.9874) (-23.5502, 17.9142) (-23.5597, 17.8226) (-23.5689, 17.7312) (-23.5778, 17.6397) (-23.5864, 17.5483) (-23.5946, 17.4569) (-23.6026, 17.3655) (-23.6102, 17.2742) (-23.6176, 17.183) (-23.6246, 17.0918) (-23.6313, 17.0006) (-23.6377, 16.9095) (-23.6438, 16.8184) (-23.6496, 16.7273) (-23.655, 16.6363) (-23.6601, 16.5454) (-23.6649, 16.4545) (-23.6693, 16.3637) (-23.6734, 16.2729) (-23.6772, 16.1821) (-23.6806, 16.0914) (-23.6837, 16.0008) (-23.6864, 15.9102) (-23.6888, 15.8197) (-23.6908, 15.7293) (-23.6925, 15.6389) (-23.6938, 15.5486) (-23.6948, 15.4583) (-23.6954, 15.3681) (-23.6956, 15.2779) (-23.6955, 15.1879) (-23.6949, 15.0979) (-23.694, 15.0079) (-23.6927, 14.9181) (-23.691, 14.8283) (-23.6889, 14.7386) (-23.6864, 14.649) (-23.6836, 14.5594) (-23.6805, 14.4773) (-23.6779, 14.4131) (-23.6758, 14.3668) (-23.6745, 14.3384) (-23.674, 14.3278) knots -1 -1 -1 -1 -1 -1 -0.985714 -0.971429 -0.957143 -0.942857 -0.928571 -0.914286 -0.9 -0.885714 -0.871429 -0.857143 -0.842857 -0.828571 -0.814286 -0.8 -0.785714 -0.771429 -0.757143 -0.742857 -0.728571 -0.714286 -0.7 -0.685714 -0.671429 -0.657143 -0.642857 -0.628571 -0.614286 -0.6 -0.585714 -0.571429 -0.557143 -0.542857 -0.528571 -0.514286 -0.5 -0.485714 -0.471429 -0.457143 -0.442857 -0.428571 -0.414286 -0.405839 -0.405839 -0.405839 -0.405839 -0.405839 -0.405839
  arc A54 (-23.674, 14.3278) -> (-24.9247, 13.9116) centre (-2.0032, -52.8695) ccw
  spline S54 degree 5 poles (-24.9247, 13.9116) (-24.9306, 13.9203) (-24.9466, 13.9439) (-24.9727, 13.9821) (-25.0091, 14.0351) (-25.0559, 14.1027) (-25.1072, 14.1761) (-25.1589, 14.2494) (-25.211, 14.3224) (-25.2635, 14.3953) (-25.3163, 14.468) (-25.3694, 14.5405) (-25.4229, 14.6129) (-25.4768, 14.6851) (-25.531, 14.7571) (-25.5855, 14.829) (-25.6404, 14.9007) (-25.6956, 14.9722) (-25.7511, 15.0436) (-25.8069, 15.1148) (-25.8631, 15.1858) (-25.9195, 15.2566) (-25.9763, 15.3274) (-26.0334, 15.3979) (-26.0908, 15.4683) (-26.1485, 15.5385) (-26.2065, 15.6086) (-26.2648, 15.6785) (-26.3234, 15.7482) (-26.3822, 15.8178) (-26.4414, 15.8872) (-26.5009, 15.9565) (-26.5606, 16.0256) (-26.6206, 16.0946) (-26.6809, 16.1634) (-26.7415, 16.2321) (-26.8023, 16.3006) (-26.8634, 16.3689) (-26.9248, 16.4371) (-26.9865, 16.5052) (-27.0484, 16.5731) (-27.1106, 16.6408) (-27.173, 16.7084) (-27.2232, 16.7623) (-27.2609, 16.8027) (-27.2861, 16.8296) (-27.2988, 16.8431) knots 0.405839 0.405839 0.405839 0.405839 0.405839 0.405839 0.414286 0.428571 0.442857 0.457143 0.471429 0.485714 0.5 0.514286 0.528571 0.542857 0.557143 0.571429 0.585714 0.6 0.614286 0.628571 0.642857 0.657143 0.671429 0.685714 0.7 0.714286 0.728571 0.742857 0.757143 0.771429 0.785714 0.8 0.814286 0.828571 0.842857 0.857143 0.871429 0.885714 0.9 0.914286 0.928571 0.942857 0.957143 0.971429 0.985714 1 1 1 1 1 1
  arc A55 (-27.2988, 16.8431) -> (-28.5381, 16.3808) centre (-2.0032, -52.8695) ccw
  spline S55 degree 5 poles (-28.5381, 16.3808) (-28.5389, 16.3624) (-28.5403, 16.3256) (-28.5424, 16.2703) (-28.545, 16.1967) (-28.5479, 16.1047) (-28.5505, 16.0128) (-28.5529, 15.9209) (-28.5549, 15.8291) (-28.5566, 15.7374) (-28.5581, 15.6457) (-28.5592, 15.5541) (-28.56, 15.4625) (-28.5605, 15.3711) (-28.5607, 15.2796) (-28.5606, 15.1883) (-28.5601, 15.097) (-28.5594, 15.0058) (-28.5583, 14.9146) (-28.5569, 14.8236) (-28.5552, 14.7326) (-28.5531, 14.6416) (-28.5507, 14.5508) (-28.548, 14.46) (-28.545, 14.3693) (-28.5416, 14.2787) (-28.5379, 14.1881) (-28.5338, 14.0977) (-28.5294, 14.0073) (-28.5246, 13.917) (-28.5195, 13.8268) (-28.514, 13.7367) (-28.5081, 13.6467) (-28.5019, 13.5568) (-28.4953, 13.467) (-28.4884, 13.3772) (-28.4811, 13.2876) (-28.4734, 13.1981) (-28.4653, 13.1086) (-28.4568, 13.0193) (-28.4479, 12.9301) (-28.4386, 12.841) (-28.4298, 12.7593) (-28.4225, 12.6954) (-28.4172, 12.6494) (-28.4139, 12.6211) (-28.4126, 12.6106) knots -1 -1 -1 -1 -1 -1 -0.985714 -0.971429 -0.957143 -0.942857 -0.928571 -0.914286 -0.9 -0.885714 -0.871429 -0.857143 -0.842857 -0.828571 -0.814286 -0.8 -0.785714 -0.771429 -0.757143 -0.742857 -0.728571 -0.714286 -0.7 -0.685714 -0.671429 -0.657143 -0.642857 -0.628571 -0.614286 -0.6 -0.585714 -0.571429 -0.557143 -0.542857 -0.528571 -0.514286 -0.5 -0.485714 -0.471429 -0.457143 -0.442857 -0.428571 -0.414286 -0.405839 -0.405839 -0.405839 -0.405839 -0.405839 -0.405839
  arc A56 (-28.4126, 12.6106) -> (-29.6304, 12.1062) centre (-2.0032, -52.8695) ccw
  spline S56 degree 5 poles (-29.6304, 12.1062) (-29.6369, 12.1145) (-29.6545, 12.1369) (-29.6833, 12.1732) (-29.7234, 12.2234) (-29.7749, 12.2875) (-29.8313, 12.3571) (-29.8881, 12.4264) (-29.9453, 12.4956) (-30.0028, 12.5646) (-30.0607, 12.6333) (-30.1189, 12.7019) (-30.1774, 12.7702) (-30.2363, 12.8384) (-30.2955, 12.9064) (-30.355, 12.9742) (-30.4148, 13.0418) (-30.475, 13.1092) (-30.5354, 13.1764) (-30.5962, 13.2434) (-30.6573, 13.3102) (-30.7187, 13.3769) (-30.7804, 13.4434) (-30.8423, 13.5097) (-30.9046, 13.5758) (-30.9672, 13.6417) (-31.03, 13.7075) (-31.0931, 13.773) (-31.1565, 13.8384) (-31.2202, 13.9036) (-31.2842, 13.9687) (-31.3484, 14.0335) (-31.4129, 14.0982) (-31.4777, 14.1627) (-31.5428, 14.227) (-31.6081, 14.2912) (-31.6737, 14.3552) (-31.7395, 14.419) (-31.8056, 14.4827) (-31.8719, 14.5461) (-31.9385, 14.6094) (-32.0054, 14.6726) (-32.0725, 14.7355) (-32.1264, 14.7858) (-32.1669, 14.8234) (-32.194, 14.8484) (-32.2075, 14.8609) knots 0.405839 0.405839 0.405839 0.405839 0.405839 0.405839 0.414286 0.428571 0.442857 0.457143 0.471429 0.485714 0.5 0.514286 0.528571 0.542857 0.557143 0.571429 0.585714 0.6 0.614286 0.628571 0.642857 0.657143 0.671429 0.685714 0.7 0.714286 0.728571 0.742857 0.757143 0.771429 0.785714 0.8 0.814286 0.828571 0.842857 0.857143 0.871429 0.885714 0.9 0.914286 0.928571 0.942857 0.957143 0.971429 0.985714 1 1 1 1 1 1
  arc A57 (-32.2075, 14.8609) -> (-33.4108, 14.3114) centre (-2.0032, -52.8695) ccw
  spline S57 degree 5 poles (-33.4108, 14.3114) (-33.4102, 14.293) (-33.409, 14.2561) (-33.4071, 14.2009) (-33.4045, 14.1272) (-33.4008, 14.0353) (-33.3969, 13.9434) (-33.3927, 13.8516) (-33.3882, 13.7599) (-33.3833, 13.6683) (-33.3782, 13.5767) (-33.3728, 13.4853) (-33.3671, 13.3939) (-33.3611, 13.3026) (-33.3547, 13.2114) (-33.3481, 13.1203) (-33.3412, 13.0293) (-33.3339, 12.9383) (-33.3263, 12.8475) (-33.3184, 12.7568) (-33.3102, 12.6661) (-33.3017, 12.5756) (-33.2928, 12.4851) (-33.2836, 12.3948) (-33.2741, 12.3045) (-33.2643, 12.2144) (-33.2541, 12.1243) (-33.2436, 12.0344) (-33.2327, 11.9446) (-33.2215, 11.8549) (-33.21, 11.7653) (-33.1981, 11.6758) (-33.1858, 11.5864) (-33.1732, 11.4972) (-33.1602, 11.408) (-33.1469, 11.319) (-33.1332, 11.2301) (-33.1191, 11.1414) (-33.1047, 11.0528) (-33.0898, 10.9643) (-33.0746, 10.8759) (-33.059, 10.7877) (-33.0443, 10.7068) (-33.0326, 10.6436) (-33.024, 10.5981) (-33.0186, 10.5702) (-33.0166, 10.5598) knots -1 -1 -1 -1 -1 -1 -0.985714 -0.971429 -0.957143 -0.942857 -0.928571 -0.914286 -0.9 -0.885714 -0.871429 -0.857143 -0.842857 -0.828571 -0.814286 -0.8 -0.785714 -0.771429 -0.757143 -0.742857 -0.728571 -0.714286 -0.7 -0.685714 -0.671429 -0.657143 -0.642857 -0.628571 -0.614286 -0.6 -0.585714 -0.571429 -0.557143 -0.542857 -0.528571 -0.514286 -0.5 -0.485714 -0.471429 -0.457143 -0.442857 -0.428571 -0.414286 -0.405839 -0.405839 -0.405839 -0.405839 -0.405839 -0.405839
  arc A58 (-33.0166, 10.5598) -> (-34.1953, 9.9698) centre (-2.0032, -52.8695) ccw
  spline S58 degree 5 poles (-34.1953, 9.9698) (-34.2024, 9.9776) (-34.2216, 9.9986) (-34.2529, 10.0328) (-34.2964, 10.0801) (-34.3524, 10.1403) (-34.4136, 10.2057) (-34.4752, 10.2708) (-34.5372, 10.3357) (-34.5995, 10.4004) (-34.6621, 10.4648) (-34.725, 10.5291) (-34.7883, 10.5931) (-34.8519, 10.6569) (-34.9158, 10.7204) (-34.98, 10.7838) (-35.0445, 10.847) (-35.1093, 10.9099) (-35.1744, 10.9726) (-35.2398, 11.0352) (-35.3055, 11.0975) (-35.3715, 11.1596) (-35.4377, 11.2215) (-35.5043, 11.2832) (-35.5711, 11.3447) (-35.6382, 11.406) (-35.7056, 11.4671) (-35.7732, 11.528) (-35.8411, 11.5887) (-35.9093, 11.6492) (-35.9778, 11.7095) (-36.0465, 11.7696) (-36.1154, 11.8295) (-36.1846, 11.8892) (-36.2541, 11.9488) (-36.3238, 12.0081) (-36.3938, 12.0672) (-36.464, 12.1262) (-36.5345, 12.185) (-36.6052, 12.2436) (-36.6762, 12.3019) (-36.7474, 12.3601) (-36.8188, 12.4182) (-36.8761, 12.4644) (-36.9192, 12.499) (-36.948, 12.5221) (-36.9624, 12.5336) knots 0.405839 0.405839 0.405839 0.405839 0.405839 0.405839 0.414286 0.428571 0.442857 0.457143 0.471429 0.485714 0.5 0.514286 0.528571 0.542857 0.557143 0.571429 0.585714 0.6 0.614286 0.628571 0.642857 0.657143 0.671429 0.685714 0.7 0.714286 0.728571 0.742857 0.757143 0.771429 0.785714 0.8 0.814286 0.828571 0.842857 0.857143 0.871429 0.885714 0.9 0.914286 0.928571 0.942857 0.957143 0.971429 0.985714 1 1 1 1 1 1
  arc A59 (-36.9624, 12.5336) -> (-38.1234, 11.8996) centre (-2.0032, -52.8695) ccw
  spline S59 degree 5 poles (-38.1234, 11.8996) (-38.1215, 11.8813) (-38.1177, 11.8446) (-38.1119, 11.7896) (-38.1039, 11.7164) (-38.0938, 11.6249) (-38.0833, 11.5336) (-38.0725, 11.4423) (-38.0615, 11.3512) (-38.0501, 11.2601) (-38.0385, 11.1692) (-38.0266, 11.0783) (-38.0144, 10.9876) (-38.0018, 10.897) (-37.989, 10.8065) (-37.9759, 10.716) (-37.9625, 10.6257) (-37.9487, 10.5356) (-37.9347, 10.4455) (-37.9204, 10.3556) (-37.9057, 10.2657) (-37.8907, 10.176) (-37.8754, 10.0864) (-37.8598, 9.997) (-37.8439, 9.9076) (-37.8276, 9.8184) (-37.8111, 9.7293) (-37.7942, 9.6404) (-37.7769, 9.5515) (-37.7593, 9.4629) (-37.7414, 9.3743) (-37.7232, 9.2859) (-37.7046, 9.1976) (-37.6856, 9.1095) (-37.6663, 9.0215) (-37.6467, 8.9337) (-37.6267, 8.846) (-37.6063, 8.7585) (-37.5856, 8.6711) (-37.5645, 8.5839) (-37.543, 8.4969) (-37.5211, 8.41) (-37.5007, 8.3304) (-37.4845, 8.2682) (-37.4726, 8.2234) (-37.4653, 8.1959) (-37.4626, 8.1857) knots -1 -1 -1 -1 -1 -1 -0.985714 -0.971429 -0.957143 -0.942857 -0.928571 -0.914286 -0.9 -0.885714 -0.871429 -0.857143 -0.842857 -0.828571 -0.814286 -0.8 -0.785714 -0.771429 -0.757143 -0.742857 -0.728571 -0.714286 -0.7 -0.685714 -0.671429 -0.657143 -0.642857 -0.628571 -0.614286 -0.6 -0.585714 -0.571429 -0.557143 -0.542857 -0.528571 -0.514286 -0.5 -0.485714 -0.471429 -0.457143 -0.442857 -0.428571 -0.414286 -0.405839 -0.405839 -0.405839 -0.405839 -0.405839 -0.405839
  arc A60 (-37.4626, 8.1857) -> (-38.5962, 7.5131) centre (-2.0032, -52.8695) ccw
  spline S60 degree 5 poles (-38.5962, 7.5131) (-38.6038, 7.5204) (-38.6245, 7.54) (-38.6581, 7.5719) (-38.7049, 7.6159) (-38.765, 7.672) (-38.8308, 7.7328) (-38.8969, 7.7934) (-38.9633, 7.8537) (-39.03, 7.9138) (-39.0971, 7.9736) (-39.1645, 8.0332) (-39.2321, 8.0925) (-39.3001, 8.1516) (-39.3684, 8.2105) (-39.4369, 8.2691) (-39.5058, 8.3275) (-39.5749, 8.3856) (-39.6443, 8.4436) (-39.714, 8.5013) (-39.784, 8.5587) (-39.8542, 8.616) (-39.9247, 8.673) (-39.9955, 8.7298) (-40.0666, 8.7864) (-40.1379, 8.8427) (-40.2094, 8.8989) (-40.2812, 8.9548) (-40.3533, 9.0105) (-40.4256, 9.066) (-40.4982, 9.1212) (-40.571, 9.1763) (-40.6441, 9.2311) (-40.7174, 9.2858) (-40.7909, 9.3402) (-40.8647, 9.3944) (-40.9387, 9.4484) (-41.013, 9.5022) (-41.0875, 9.5558) (-41.1622, 9.6092) (-41.2371, 9.6624) (-41.3123, 9.7153) (-41.3876, 9.7681) (-41.4481, 9.8101) (-41.4936, 9.8416) (-41.524, 9.8625) (-41.5391, 9.873) knots 0.405839 0.405839 0.405839 0.405839 0.405839 0.405839 0.414286 0.428571 0.442857 0.457143 0.471429 0.485714 0.5 0.514286 0.528571 0.542857 0.557143 0.571429 0.585714 0.6 0.614286 0.628571 0.642857 0.657143 0.671429 0.685714 0.7 0.714286 0.728571 0.742857 0.757143 0.771429 0.785714 0.8 0.814286 0.828571 0.842857 0.857143 0.871429 0.885714 0.9 0.914286 0.928571 0.942857 0.957143 0.971429 0.985714 1 1 1 1 1 1
  arc A61 (-41.5391, 9.873) -> (-42.6519, 9.1578) centre (-2.0032, -52.8695) ccw
  spline S61 degree 5 poles (-42.6519, 9.1578) (-42.6487, 9.1397) (-42.6423, 9.1034) (-42.6326, 9.0489) (-42.6195, 8.9764) (-42.6028, 8.886) (-42.5858, 8.7956) (-42.5686, 8.7053) (-42.5511, 8.6152) (-42.5332, 8.5252) (-42.5152, 8.4353) (-42.4968, 8.3455) (-42.4781, 8.2559) (-42.4592, 8.1664) (-42.4399, 8.077) (-42.4204, 7.9878) (-42.4005, 7.8987) (-42.3804, 7.8097) (-42.36, 7.7209) (-42.3393, 7.6322) (-42.3182, 7.5436) (-42.2969, 7.4552) (-42.2753, 7.3669) (-42.2533, 7.2788) (-42.231, 7.1908) (-42.2085, 7.103) (-42.1856, 7.0153) (-42.1624, 6.9278) (-42.1388, 6.8404) (-42.115, 6.7532) (-42.0908, 6.6662) (-42.0663, 6.5793) (-42.0414, 6.4926) (-42.0163, 6.406) (-41.9907, 6.3197) (-41.9649, 6.2335) (-41.9387, 6.1474) (-41.9121, 6.0616) (-41.8852, 5.9759) (-41.8579, 5.8904) (-41.8303, 5.8051) (-41.8023, 5.72) (-41.7762, 5.6421) (-41.7556, 5.5812) (-41.7406, 5.5374) (-41.7313, 5.5105) (-41.7279, 5.5005) knots -1 -1 -1 -1 -1 -1 -0.985714 -0.971429 -0.957143 -0.942857 -0.928571 -0.914286 -0.9 -0.885714 -0.871429 -0.857143 -0.842857 -0.828571 -0.814286 -0.8 -0.785714 -0.771429 -0.757143 -0.742857 -0.728571 -0.714286 -0.7 -0.685714 -0.671429 -0.657143 -0.642857 -0.628571 -0.614286 -0.6 -0.585714 -0.571429 -0.557143 -0.542857 -0.528571 -0.514286 -0.5 -0.485714 -0.471429 -0.457143 -0.442857 -0.428571 -0.414286 -0.405839 -0.405839 -0.405839 -0.405839 -0.405839 -0.405839
  arc A62 (-41.7279, 5.5005) -> (-42.8106, 4.7487) centre (-2.0032, -52.8695) ccw